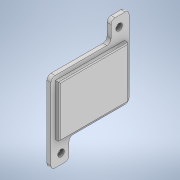
# Autodesk Inventor part: deckel_wemos
Saved by Autodesk Inventor 2020 (Build 240168000, 168)
## iProperties
Created: 2020-05-23
Part Number: deckel_wemos
Material: Generisch
Document SubType Name: Modeling
Designer: chris
Density: 1 g/cm^3
Appearance: Vorgabe
Author: chris
Autodesk Inventor part; units mm, degrees
ref_plane "YZ Plane" through (0, 0, 0) normal (1, 0, 0) x (0, 1, 0)
ref_plane "XZ Plane" through (0, 0, 0) normal (0, 1, 0) x (-1, 0, 0)
ref_plane "XY Plane" through (0, 0, 0) normal (0, 0, 1) x (1, 0, 0)
sketch "Skizze1" plane through (0, 0, 0) normal (1, 0, 0) x (0, 1, 0)
  line L0 (0, 0) -> (30, 0)
  line L1 (30, 0) -> (30, -39)
  line L2 (30, -39) -> (0, -39)
  line L3 (0, -39) -> (0, 0)
  dimension "d0" = 30
  dimension "d1" = 39
  constraints: 8 end point, 2 parallel, 1 horizontal, 1 perpendicular
  measures "d0" distance of L0.start L0.end
  measures "d1" distance between parallel lines of L2 L0
extrude "Extrusion1" add sketch "Skizze1" along normal blind 2
sketch "Skizze2" plane through (2, 0, 0) normal (1, 0, 0) x (0, 0, -1)
  line L0 (2.2, 27.8) -> (36.8, 27.8)
  line L1 (36.8, 27.8) -> (36.8, 2.2)
  line L2 (36.8, 2.2) -> (2.2, 2.2)
  line L3 (2.2, 2.2) -> (2.2, 27.8)
  line L4 (0, 30) -> (0, 0) projected
  line L5 (39, 30) -> (0, 30) projected
  dimension "d4" = 25.6
  dimension "d5" = 34.6
  dimension "d6" = 2.2
  dimension "d7" = 2.2
  constraints: 8 end point, 2 parallel, 1 horizontal, 1 perpendicular
  measures "d4" distance between parallel lines of L2 L0
  measures "d5" distance between parallel lines of L1 L3
  measures "d6" distance between parallel lines of L4 L3
  measures "d7" distance between parallel lines of L5 L0
extrude "Extrusion2" add sketch "Skizze2" along normal blind 2
chamfer "Fase1" distance 0.5 angle 45 4 edges at (4, 27.8, -19.5) (4, 15, -2.2) (4, 2.2, -19.5) (4, 15, -36.8)
sketch "Skizze3" plane through (0, 0, 0) normal (-1, 0, 0) x (0, 0, 1)
  line L0 (0, 0) -> (-39, 0) projected
  line L1 (0, 0) -> (-9, 0)
  line L2 (-9, 0) -> (-9, -10)
  line L3 (-9, -10) -> (0, -10)
  line L4 (0, -10) -> (0, 0)
  line L5 (-39, 0) -> (-39, 30) projected
  line L6 (-39, 30) -> (-30, 30)
  line L7 (-30, 30) -> (-30, 40)
  line L8 (-30, 40) -> (-39, 40)
  line L9 (-39, 40) -> (-39, 30)
  circle A0 centre (-5, -5) radius 1.65
  circle A1 centre (-34, 35) radius 1.65
  dimension "d13" = 10
  dimension "d14" = 9
  dimension "d15" = 9
  dimension "d16" = 10
  dimension "d17" = 5
  dimension "d18" = 5
  dimension "d19" = 3.3
  dimension "d20" = 5
  dimension "d21" = 5
  dimension "d22" = 3.3
  constraints: 16 end point, 4 parallel, 2 centre point, 2 horizontal, 2 perpendicular
  measures "d13" distance between parallel lines of L0 L3
  measures "d14" distance between parallel lines of L2 L4
  measures "d15" distance between parallel lines of L9 L7
  measures "d16" distance between parallel lines of L6 L8
  measures "d17" distance from line of L4 A0.centre
  measures "d18" distance from line of L3 A0.centre
  measures "d19" diameter of A0
  measures "d20" distance from line of L9 A1.centre
  measures "d21" distance from line of L8 A1.centre
  measures "d22" diameter of A1
extrude "Extrusion3" add sketch "Skizze3" against normal blind 2
fillet "Rundung1" radius 2 8 edges at (1, -10, 0) (1, -10, -9) (1, 0, -39) (1, 40, -39) (1, 0, -9) (1, 40, -30) (1, 30, -30) (1, 30, 0)
